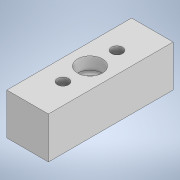
# Autodesk Inventor part: LoadCellUpperPiece
Saved by Autodesk Inventor 2022 (Build 260153000, 153)
## iProperties
Created: 2021-11-03
Part Number: LoadCellUpperPiece
Material: Genérico
Document SubType Name: Modeling
Designer: JK
Density: 1 g/cm^3
Appearance: Valor por defecto
Author: JK
Autodesk Inventor part; units mm, degrees
ref_plane "YZ Plane" through (0, 0, 0) normal (1, 0, 0) x (0, 1, 0)
ref_plane "XZ Plane" through (0, 0, 0) normal (0, 1, 0) x (-1, 0, 0)
ref_plane "XY Plane" through (0, 0, 0) normal (0, 0, 1) x (1, 0, 0)
sketch "Boceto1" plane through (0, 0, 0) normal (0, 1, 0) x (-1, 0, 0)
  line L0 (-10, 30) -> (10, 30)
  line L1 (10, 30) -> (10, -30)
  line L2 (10, -30) -> (-10, -30)
  line L3 (-10, -30) -> (-10, 30)
  line L4 (-10, 30) -> (10, -30) construction
  line L5 (10, 30) -> (-10, -30) construction
  circle A0 centre (0, 0) radius 3
  dimension "d0" = 6
  dimension "d1" = 60
  dimension "d2" = 20
  constraints: 12 end point, 2 midpoint, 2 parallel, 1 centre point, 1 coincident, 1 horizontal, 1 perpendicular
  measures "d0" diameter of A0
  measures "d1" distance of L0.end L1.end
  measures "d2" distance of L1.end L2.end
extrude "Extrusión1" add sketch "Boceto1" along normal blind 10
sketch "Boceto2" plane through (0, 0, 0) normal (0, -1, 0) x (1, 0, 0)
  circle A0 centre (0, 13) radius 2.7
  circle A1 centre (0, -13) radius 2.7
  point P0 (0, 0)
  dimension "d5" = 5.4
  dimension "d6" = 13
  dimension "d7" = 13
  constraints: 2 centre point, 1 equal radius
  measures "d5" diameter of A0
  measures "d6" distance of point (0, 0) A0.centre
  measures "d7" distance of point (0, 0) A1.centre
extrude "Extrusión2" cut sketch "Boceto2" against normal through all
sketch "Boceto3" plane through (0, 0, 0) normal (0, -1, 0) x (1, 0, 0)
  line L0 (-6.5, 25.5) -> (6.5, 25.5)
  line L1 (6.5, 25.5) -> (6.5, -25.5)
  line L2 (6.5, -25.5) -> (-6.5, -25.5)
  line L3 (-6.5, -25.5) -> (-6.5, 25.5)
  circle A0 centre (0, 0) radius 3 projected
  line L4 (-6.5, 25.5) -> (6.5, -25.5) construction
  line L5 (6.5, 25.5) -> (-6.5, -25.5) construction
  circle A1 centre (0, -13) radius 2.7 projected
  circle A2 centre (0, 13) radius 2.7 projected
  line L6 (10, -30) -> (-10, -30) projected
  line L7 (10, 30) -> (10, -30) projected
  line L8 (-10, 30) -> (10, 30) projected
  line L9 (-10, -30) -> (-10, 30) projected
  circle A3 centre (0, 0) radius 3 projected
  dimension "d10" = 51
  dimension "d11" = 13
  constraints: 12 end point, 2 midpoint, 2 parallel, 1 horizontal, 1 perpendicular
  measures "d10" distance of L0.end L1.end
  measures "d11" distance of L1.end L2.end
extrude "Extrusión3" add sketch "Boceto3" along normal blind 10 contours L6 L9 L8 L7
sketch "Boceto4" plane through (0, 10, 0) normal (0, 1, 0) x (1, 0, 0)
  circle A0 centre (0, 0) radius 6
  dimension "d14" = 12
  constraints: 1 centre point, 1 coincident
  measures "d14" diameter of A0
extrude "Extrusión4" cut sketch "Boceto4" against normal blind 6
